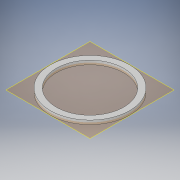
# Autodesk Inventor part: FRA_015_TurntableBeltPulleyMockup
Saved by Autodesk Inventor 2018 (Build 220112000, 112)
## iProperties
Created: 2020-01-26
Part Number: FRA_015_TurntableBeltPulleyMockup
Material: Generic
Document SubType Name: Modeling
Designer: 22barlalex
Density: 1 g/cm^3
Appearance: Default
Author: 22barlalex
Autodesk Inventor part; units mm, degrees
ref_plane "YZ Plane" through (0, 0, 0) normal (1, 0, 0) x (0, 1, 0)
ref_plane "XZ Plane" through (0, 0, 0) normal (0, 1, 0) x (-1, 0, 0)
ref_plane "XY Plane" through (0, 0, 0) normal (0, 0, 1) x (1, 0, 0)
sketch "Sketch1" plane through (0, 0, 0) normal (0, 1, 0) x (-1, 0, 0)
  circle A0 centre (0, 0) radius 162.56
  circle A1 centre (0, 0) radius 191.008
  dimension "d0" = 325.12
  dimension "d1" = 382.016
  constraints: 2 centre point, 2 coincident
  measures "d0" diameter of A0
  measures "d1" diameter of A1
extrude "Extrusion1" add sketch "Sketch1" along normal blind 19.05
ref_plane "Work Plane1" through (0, 9.525, 0) normal (0, 1, 0) x (1, 0, 0)
body "Solid1"
